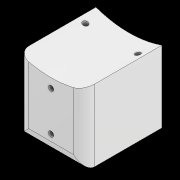
# Autodesk Inventor part: AttatchmentUpper
Saved by Autodesk Inventor 2022.2 (Build 262287010, 287A)
## iProperties
Created: 2022-04-29
Part Number: AttatchmentUpper
Material: ABS Plastic
Document SubType Name: Modeling
Designer: Árni Þór Þorgeirsson
Density: 1.06 g/cm^3
Appearance: Smooth - White
Mass: 499.111 g
Surface Area: 672.501 cm^2
Volume: 499.111 cm^3
Author: Árni Þór Þorgeirsson
Autodesk Inventor part; units mm, degrees
ref_plane "YZ Plane" through (0, 0, 0) normal (1, 0, 0) x (0, 1, 0)
ref_plane "XZ Plane" through (0, 0, 0) normal (0, 1, 0) x (-1, 0, 0)
sketch "Sketch3" plane through (0, 0, 0) normal (0, 1, 0) x (-1, 0, 0)
  line L0 (0, 0) -> (0, 31.5556)
  constraints: 2 end point, 1 vertical
sketch "Sketch1" plane through (0, 0, 0) normal (0, 0, 1) x (1, 0, 0)
  circle A0 centre (0, 0) radius 75
  circle A1 centre (63.483, 20.6269) radius 6 construction
  circle A2 centre (-63.483, -20.6269) radius 6 construction
  circle A3 centre (0, 0) radius 69 construction
  line L0 (0, 0) -> (0.0001, -211.0949) construction
  arc A4 (-59.7327, 15.2299) -> (-60.2661, -15.5622) centre (-48.002, -0.374) ccw construction
  line L1 (0.2505, 0.4177) -> (-45.224, -139.5383) construction
  line L2 (-0.1358, 0.4177) -> (49.2707, -151.6398) construction
  line L3 (0, 0) -> (0.0001, -82)
  line L4 (0.0001, -82) -> (0.0001, -112)
  circle A5 centre (0.0001, -82) radius 2
  circle A6 centre (0.0001, -112) radius 2
  line L5 (0.0001, -82) -> (25.0001, -82)
  line L6 (0.0001, -82) -> (-24.9999, -82)
  line L7 (25.0001, -112) -> (25.0001, -70.7106)
  line L8 (-24.9999, -112) -> (-24.9999, -70.7107)
  line L9 (25.0001, -125) -> (25.0001, -112)
  line L10 (25.0001, -125) -> (-24.9999, -125)
  line L11 (-24.9999, -125) -> (-24.9999, -112)
  point P0 (56.6452, 18.2098)
  point P1 (56.6452, 18.2098)
  point P2 (57.7767, 18.7728)
  point P3 (56.6452, 18.2098)
  point P4 (57.7767, 18.7728)
  point P5 (56.6794, 18.5913)
  point P6 (-19.8743, -61.5198)
  point P7 (19.9889, -61.5198)
  point P8 (19.9889, -61.5198)
  point P9 (0.0001, -75)
  dimension "d19" = 12
  dimension "d66" = 12
  dimension "d4" = 150
  dimension "d59" = 66.75
  dimension "d67" = 63.483
  dimension "d68" = 138
  dimension "d147" = 18
  dimension "d148" = 18
  dimension "d157" = 82
  dimension "d158" = 30
  dimension "d159" = 4
  dimension "d160" = 4
  dimension "d161" = 25
  dimension "d162" = 25
  dimension "d163" = 25
  dimension "d164" = 25
  dimension "d165" = 50
  constraints: 24 end point, 8 coincident, 5 centre point, 5 point on circle, 5 point on line, 3 horizontal, 2 vertical, 1 collinear, 1 perpendicular, 12 other
  measures "d4" diameter of A0
  measures "d59" distance of point (63.483, 20.627) A0.centre
  measures "d67" horizontal distance of A0.centre point (-63.483, -20.627)
  measures "d68" diameter of A3
  measures "d147" angle of L0 L1
  measures "d148" angle of L0 L2
  measures "d157" distance of L3.start L3.end
  measures "d158" distance of L3.end L4.end
  measures "d159" diameter of A5
  measures "d160" diameter of A6
  measures "d161" distance of L5.start L5.end
  measures "d162" distance of L5.start L6.end
  measures "d163" distance of A6.centre L8.start
  measures "d164" distance of A6.centre L7.start
  measures "d165" distance from line of L10 point (0, -75)
ref_plane "Work Plane1" through (0, 0, 100) normal (0, 0, 1) x (1, 0, 0)
sketch "Sketch9" plane through (0, 0, 100) normal (0, 0, 1) x (1, 0, 0)
  circle A0 centre (0, 0) radius 75
  spline S0 degree 3 number of poles 235
  circle A1 centre (0, 0) radius 69
  line L0 (0, -270.1399) -> (0, 140.0417) construction
  line L1 (-118.2892, 0) -> (124.185, 0) construction
  point P0 (0, 0)
  point P1 (59.5, 0)
  point P2 (69, 0)
  dimension "d112" = 69
  constraints: 1 coincident, 1 horizontal alignment, 1 point on line, 2 other
extrude "Extrusion7" [suppressed]
sketch "Sketch10" plane through (0, 0, 2.5) normal (0, 0, 1) x (1, 0, 0)
  circle A0 centre (69, 0) radius 1.5
  line L0 (71.75, -1.5877) -> (69, -3.1754)
  line L1 (69, -3.1754) -> (66.25, -1.5877)
  line L2 (66.25, -1.5877) -> (66.25, 1.5877)
  line L3 (66.25, 1.5877) -> (69, 3.1754)
  line L4 (69, 3.1754) -> (71.75, 1.5877)
  line L5 (71.75, 1.5877) -> (71.75, -1.5877)
  point P0 (0, 0)
  dimension "d115" = 3
  dimension "d118" = 5.5
  constraints: 12 end point, 2 coincident, 1 centre point, 13 other
  measures "d115" diameter of A0
  measures "d118" distance between parallel lines of L5 L2
extrude "Extrusion10" [suppressed]
pattern_circular "Circular Pattern4" [suppressed]
extrude "Extrusion8" [suppressed]
extrude "Extrusion9" [suppressed]
pattern_circular "Circular Pattern3" [suppressed]
extrude "Extrusion3" [suppressed]
sketch "Sketch12" plane through (0, 0, -13.15) normal (0, 0, -1) x (-1, 0, 0)
  circle A0 centre (0, 0) radius 69
  point P0 (-65.6229, -21.3222)
  dimension "d132" = 138
  constraints: 1 coincident, 3 other
hole "Hole3" [suppressed]
pattern_circular "Circular Pattern5" [suppressed]
sketch "Sketch13" plane through (0, 0, 0) normal (0, 1, 0) x (-1, 0, 0)
  line L0 (-64.5572, 13.15) -> (64.4426, 13.15) projected
  line L1 (-64.5572, -13.15) -> (64.4426, -13.15) projected
  line L2 (75, 13.15) -> (-75, 13.15) projected
  line L3 (-23.4889, 2.0207) -> (-19.9889, 4.0415)
  line L4 (-19.9889, 4.0415) -> (-16.4889, 2.0207)
  line L5 (-16.4889, 2.0207) -> (-16.4889, -2.0207)
  line L6 (-16.4889, -2.0207) -> (-19.9889, -4.0415)
  line L7 (-19.9889, -4.0415) -> (-23.4889, -2.0207)
  line L8 (-23.4889, -2.0207) -> (-23.4889, 2.0207)
  line L9 (16.3743, 2.0207) -> (19.8743, 4.0415)
  line L10 (19.8743, 4.0415) -> (23.3743, 2.0207)
  line L11 (23.3743, 2.0207) -> (23.3743, -2.0207)
  line L12 (23.3743, -2.0207) -> (19.8743, -4.0415)
  line L13 (19.8743, -4.0415) -> (16.3743, -2.0207)
  line L14 (16.3743, -2.0207) -> (16.3743, 2.0207)
  circle A0 centre (19.8743, 0) radius 2
  circle A1 centre (-19.9889, 0) radius 2
  point P0 (0, 0)
  point P1 (-56.6452, 13.15)
  point P2 (-56.6452, -13.15)
  dimension "d149" = 7
  dimension "d150" = 7
  dimension "d153" = 4
  dimension "d154" = 4
  constraints: 24 end point, 4 coincident, 2 centre point, 26 other
  measures "d149" distance between parallel lines of L5 L8
  measures "d150" distance from line of L11.end L14
  measures "d153" diameter of A0
  measures "d154" diameter of A1
extrude "Extrusion12" [suppressed]
extrude "Extrusion13" [suppressed]
extrude "Extrusion14" add sketch "Sketch1" along normal mid plane 26.3 contours A0 L3 A5 L6 L8 | L7 L5 A5 L3 A0 | L6 A5 L5 L7 L9 L10 L11 L8
sketch "Sketch14" plane through (-24.9999, -125, 13.15) normal (0, -1, 0) x (1, 0, 0)
  circle A0 centre (5.1257, -13.15) radius 2 projected
  line L0 (8.6257, -11.1293) -> (5.1257, -9.1085) projected
  line L1 (5.1257, -9.1085) -> (1.6257, -11.1293) projected
  line L2 (1.6257, -11.1293) -> (1.6257, -15.1707) projected
  line L3 (1.6257, -15.1707) -> (5.1257, -17.1915) projected
  line L4 (5.1257, -17.1915) -> (8.6257, -15.1707) projected
  line L5 (8.6257, -15.1707) -> (8.6257, -11.1293) projected
  line L6 (44.9889, -9.1085) -> (41.4889, -11.1293) projected
  circle A1 centre (44.9889, -13.15) radius 2 projected
  line L7 (48.4889, -11.1293) -> (44.9889, -9.1085) projected
  line L8 (48.4889, -15.1707) -> (48.4889, -11.1293) projected
  line L9 (44.9889, -17.1915) -> (48.4889, -15.1707) projected
  line L10 (41.4889, -15.1707) -> (44.9889, -17.1915) projected
  line L11 (41.4889, -11.1293) -> (41.4889, -15.1707) projected
  point P0 (24.9999, -13.15)
extrude "Extrusion15" cut sketch "Sketch14" against normal through all contours A0 | A1
extrude "Extrusion16" cut sketch "Sketch14" against normal blind 4 contours A0 | L5 L4 L3 L2 L1 L0 | L7 L8 L9 L10 L11 L6 | A1
sketch "Sketch15" plane through (0, 0, 13.15) normal (0, 0, 1) x (1, 0, 0)
  line L0 (-24.9999, -70.7107) -> (-24.9999, -125) projected
  line L1 (-24.9999, -125) -> (25.0001, -125) projected
  line L2 (25.0001, -125) -> (25.0001, -70.7106) projected
  arc A0 (-24.9999, -70.7107) -> (25.0001, -70.7106) centre (0, 0) ccw projected
  circle A1 centre (0.0001, -82) radius 2 projected
  circle A2 centre (0.0001, -112) radius 2 projected
  point P0 (0, 0)
  dimension "d99" = 156
extrude "Extrusion17" add sketch "Sketch15" along normal blind 32.694
fillet "Fillet2" radius 8 3 edges at (25.0001, -97.8553, 45.844) (-24.9999, -97.8554, 45.844) (0.0001, -125, 45.844)
sketch "Sketch8" plane through (0, 0, -13.15) normal (0, 0, -1) x (-1, 0, 0)
  circle A0 centre (0, 0) radius 78 projected
  arc A1 (-23.65, -105.9607) -> (-46.4722, -58.8671) centre (-83.65, -105.9607) ccw projected
  arc A2 (46.4722, -58.8671) -> (23.65, -105.9607) centre (83.65, -105.9607) ccw projected
  line L0 (23.65, -200) -> (23.65, -105.9607) projected
  line L1 (-23.65, -105.9607) -> (-23.65, -200) projected
  arc A3 (-23.65, -200) -> (23.65, -200) centre (0, -181.5425) ccw projected
  point P0 (36.3948, -68.9886)
  point P1 (-36.3948, -68.9886)
sketch "Sketch11" plane through (0, 0, 2.5) normal (0, 0, 1) x (1, 0, 0)
  circle A0 centre (0, 0) radius 11.25
  dimension "d129" = 22.5
  constraints: 1 centre point, 1 coincident
  measures "d129" diameter of A0
equation "\"Axle_diameter\" = 6"
equation "\"Compensation\" = 0.45"
equation "\"Bearing_Outer_Hole_Location\" = 138"
equation "\"Printer_Gap_Fit\" = 0.1"
equation "\"Printer_Gap_Slide\" = 0.3"
equation "\"Bearing_Roller_Diameter\" = 8"
equation "\"Fastners_ScrewHeadThickness\" = 2"
equation "\"Fastners_OuterThicknessFromScrew\" = 5"
equation "\"Fastners_InnerThicknessFromScrew\" = 2"
equation "\"Fastners_OutputAxisHeadThickness\" = 2"
equation "\"Printer_HoleCompensation\" = 0"
equation "\"Bearing_Outer_Radius\" = 75"
equation "\"Bearing_Thicness_compensation\" = 0.27244"
equation "\"Bearing_To_12mm\" = 0.27244"
equation "\"Bearing_Inner_Hole_Location\" = 84"
equation "\"Housing_Outer_Hole_Location\" = 138"
equation "\"Bearing_Gap_Fit\" = 0.1"
equation "\"Bearing_Gap_Slide\" = 0.43"
equation "\"Bearing_ScrewHeadThickness\" = 2"
equation "\"Bearing_OuterThicknessFromScrew\" = 5"
equation "\"Bearing_InnerThicknessFromScrew\" = 2"
equation "\"Bearing_OutputAxisHeadThickness\" = 2"
equation "\"Bearing_HoleCompensation\" = 0.5"
equation "\"Roller_radius\" = 5"
equation "\"Pin_set_dimention\" = 22"
equation "\"Pin_bearing_outer_dimention\" = 22"
equation "\"Shaft_dimention\" = 2"
equation "\"Pin_bearing_inner_dimention\" = 3"
equation "\"Rotor_dimention\" = 125"
equation "\"Rotor_radius\" = 62.5"
equation "\"Outer_rotor_radius\" = 65"
equation "\"Output_hole_set_diameter\" = 24.5"
equation "\"Bearing_ScrewDiameter\" = 3.5"
equation "\"Bearing_ScrewHeadDiameter\" = 5.5"
equation "\"Bearing_OutputAxisHeadDiameter\" = 8.5"
equation "\"BearingHoleThrough\" = 12"
equation "\"Fastners_ScrewDiameter\" = 3"
equation "\"Bearing_OutputAxisDiameter\" = 6"
equation "\"Fastners_ScrewHeadDiameter\" = 5"
equation "\"Fastners_OutputAxisHeadDiameter\" = 12"
equation "\"BraceMountThickness\" = 47.3"
equation "\"R\" = 1"
equation "\"Rr\" = 1"
equation "\"Ece\" = 1"
equation "\"Num\" = 1"
equation "\"formula\" = 1"
body "Solid2"
body "Solid3"
